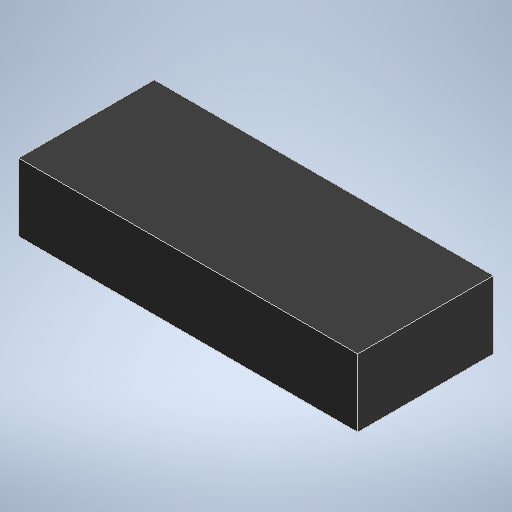
# Autodesk Inventor part: E Component 2
Saved by Autodesk Inventor 2026.2 (Build 302298010, 298A)
## iProperties
Created: 2026-05-02
Part Number: E Component 2
Material: Rubber, Silicone
Document SubType Name: Modeling
Designer: piete
Density: 1.25 g/cm^3
Appearance: Rubber - Black
Author: piete
Autodesk Inventor part; units mm, degrees
ref_plane "YZ Plane" through (0, 0, 0) normal (1, 0, 0) x (0, 1, 0)
ref_plane "XZ Plane" through (0, 0, 0) normal (0, 1, 0) x (-1, 0, 0)
ref_plane "XY Plane" through (0, 0, 0) normal (0, 0, 1) x (1, 0, 0)
sketch "Sketch1" plane through (0, 0, 0) normal (0, 1, 0) x (-1, 0, 0)
  line L0 (2.5, 1) -> (-2.5, 1)
  line L1 (-2.5, 1) -> (-2.5, -1)
  line L2 (-2.5, -1) -> (2.5, -1)
  line L3 (2.5, -1) -> (2.5, 1)
  point P0 (0, 0)
  dimension "d0" = 5
  dimension "d1" = 2
  dimension "d2" = 2.5
  dimension "d3" = 1
  constraints: 8 end point, 2 parallel, 1 horizontal, 1 perpendicular
  measures "d0" distance of L2.end L1.end
  measures "d1" distance of L1.end L0.end
  measures "d2" distance from line of point (0, 0) L3
  measures "d3" distance from line of L0 point (0, 0)
extrude "Extrusion1" add sketch "Sketch1" along normal blind 1
equation "\"d2\" = 0.5 * d0"
equation "\"d3\" = 0.5 * d1"
body "Solid1"
